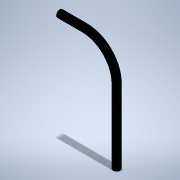
# Autodesk Inventor part: 1216.1001_LightPipe
Saved by Autodesk Inventor 2022.2 (Build 262287010, 287A)
## iProperties
Created: 2022-03-29
Part Number: 1216.1001_LightPipe
Material: Generic
Document SubType Name: Modeling
Designer: Graeme
Density: 1 g/cm^3
Appearance: Default
Author: Graeme
Autodesk Inventor part; units mm, degrees
ref_plane "YZ Plane" through (0, 0, 0) normal (1, 0, 0) x (0, 1, 0)
ref_plane "XZ Plane" through (0, 0, 0) normal (0, 1, 0) x (-1, 0, 0)
ref_plane "XY Plane" through (0, 0, 0) normal (0, 0, 1) x (1, 0, 0)
sketch "Sketch1" plane through (0, 0, 0) normal (0, 0, 1) x (1, 0, 0)
  line L0 (-4.802, -34.53) -> (1.598, -34.53)
  line L1 (-4.802, -32.53) -> (1.598, -32.53)
  line L2 (-4.802, -37.03) -> (-4.802, -30.03) projected
  line L3 (9.9692, -58.5748) -> (10.8192, -58.5748) projected
  line L4 (11.3192, -58.5748) -> (12.1692, -58.5748) projected
  line L5 (12.8442, -63.0748) -> (9.2942, -63.0748) projected
  line L6 (-4.802, -33.53) -> (11.0692, -33.53) construction
  line L7 (11.0692, -63.0748) -> (11.0692, -33.53) construction
  circle A0 centre (2.0692, -42.53) radius 9 construction
  arc A1 (11.0692, -42.53) -> (2.0692, -33.53) centre (2.0692, -42.53) ccw
  line L8 (2.0692, -33.53) -> (-4.802, -33.53)
  line L9 (11.0692, -63.0748) -> (11.0692, -42.53)
  point P0 (0, 0)
  dimension "d0" = 18
  constraints: 13 end point, 5 horizontal, 2 collinear, 2 midpoint, 2 point on circle, 2 vertical, 1 centre point, 1 coincident, 1 perpendicular, 1 point on line, 1 vertical alignment, 6 other
sketch "Sketch2" plane through (0, 0, 0) normal (1, 0, 0) x (0, 1, 0)
  circle A0 centre (-33.53, 0) radius 1 projected
  circle A1 centre (-33.53, 0) radius 1
  point P0 (0, 0)
  constraints: 1 centre point, 1 coincident, 1 concentric
sweep "Sweep1" add profiles "Sketch2" path "Sketch1" path curves L8 A1 L9
body "Solid1"
